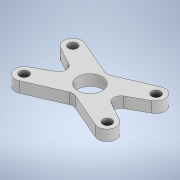
# Autodesk Inventor part: Extension2
Saved by Autodesk Inventor 2021 (Build 250183000, 183)
## iProperties
Created: 2021-04-02
Part Number: Extension2
Material: Genérico
Document SubType Name: Modeling
Designer: diego
Density: 1 g/cm^3
Appearance: Valor por defecto
Author: diego
Autodesk Inventor part; units mm, degrees
ref_plane "YZ Plane" through (0, 0, 0) normal (1, 0, 0) x (0, 1, 0)
ref_plane "XZ Plane" through (0, 0, 0) normal (0, 1, 0) x (-1, 0, 0)
ref_plane "XY Plane" through (0, 0, 0) normal (0, 0, 1) x (1, 0, 0)
sketch "Boceto1" plane through (0, 0, 0) normal (0, 1, 0) x (-1, 0, 0)
  arc A0 (22.0076, -15.7946) -> (23.9924, -11.2054) centre (23, -13.5) ccw
  arc A1 (23.9924, -2.2946) -> (22.0076, 2.2946) centre (23, 0) ccw
  arc A2 (0.9924, 2.2946) -> (-0.9924, -2.2946) centre (0, 0) ccw
  arc A3 (-0.9924, -11.2054) -> (0.9924, -15.7946) centre (0, -13.5) ccw
  line L0 (12.2939, -1.9066) -> (22.0076, 2.2946)
  line L1 (19.1337, -5.0031) -> (23.9924, -2.2946)
  line L2 (19.1337, -8.4969) -> (23.9924, -11.2054)
  line L3 (0.9924, 2.2946) -> (10.7061, -1.9066)
  line L4 (-0.9924, -2.2946) -> (3.8663, -5.0031)
  line L5 (3.8663, -8.4969) -> (-0.9924, -11.2054)
  line L6 (12.2939, -11.5934) -> (22.0076, -15.7946)
  line L7 (10.7061, -11.5934) -> (0.9924, -15.7946)
  circle A4 centre (11.5, -6.75) radius 3.4
  arc A5 (19.1337, -5.0031) -> (19.1337, -8.4969) centre (20.1075, -6.75) ccw
  arc A6 (10.7061, -1.9066) -> (12.2939, -1.9066) centre (11.5, -0.071) ccw
  arc A7 (3.8663, -8.4969) -> (3.8663, -5.0031) centre (2.8925, -6.75) ccw
  arc A8 (12.2939, -11.5934) -> (10.7061, -11.5934) centre (11.5, -13.429) ccw
  circle A9 centre (23, 0) radius 1.25
  circle A10 centre (23, -13.5) radius 1.25
  circle A11 centre (-0.0735, 0) radius 1.25
  circle A12 centre (-0.0735, -13.5) radius 1.25
  constraints: 16 end point, 16 point on circle, 13 centre point, 10 tangent, 3 coincident, 3 equal radius
extrude "Extrusión1" add sketch "Boceto1" along normal blind 3
